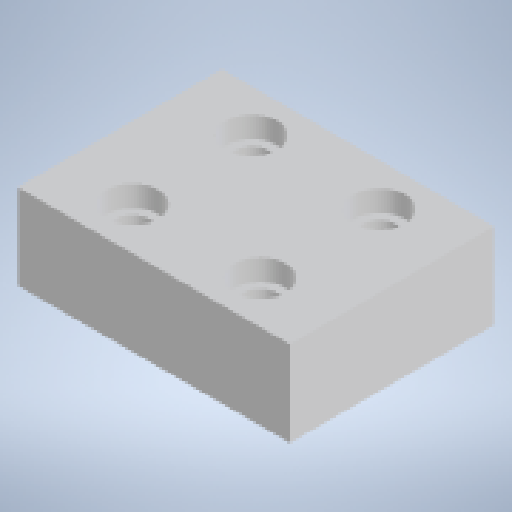
# Autodesk Inventor part: WristMotorTensioner
Saved by Autodesk Inventor 2024 (Build 280153000, 153)
## iProperties
Created: 2024-02-06
Part Number: WristMotorTensioner
Material: Generic
Document SubType Name: Modeling
Designer: Irwin
Density: 1 g/cm^3
Appearance: Default
Author: Irwin
Autodesk Inventor part; units mm, degrees
ref_plane "YZ Plane" through (0, 0, 0) normal (1, 0, 0) x (0, 1, 0)
ref_plane "XZ Plane" through (0, 0, 0) normal (0, 1, 0) x (-1, 0, 0)
ref_plane "XY Plane" through (0, 0, 0) normal (0, 0, 1) x (1, 0, 0)
sketch "Sketch1" plane through (0, 0, 0) normal (0, 1, 0) x (-1, 0, 0)
  line L0 (0, 0) -> (-32, 0)
  line L1 (-32, 0) -> (-32, -24)
  line L2 (-32, -24) -> (0, -24)
  line L3 (0, -24) -> (0, 0)
  circle A0 centre (-8.5, -19) radius 2
  circle A1 centre (-23.5, -19) radius 2
  circle A2 centre (-23.5, -5) radius 2
  circle A3 centre (-8.5, -5) radius 2
  line L4 (-16, -24) -> (-16, 0) construction
  line L5 (0, -12) -> (-32, -12) construction
  dimension "d0" = 32
  dimension "d1" = 24
  dimension "x" = 4
  dimension "d3" = 4
  dimension "d4" = 4
  dimension "d5" = 4
  dimension "d6" = 15
  dimension "d7" = 7.5
  dimension "d8" = 14
  dimension "d9" = 7
  constraints: 12 end point, 4 centre point, 4 midpoint, 2 horizontal alignment, 2 parallel, 2 vertical alignment, 1 horizontal, 1 perpendicular
  measures "d0" distance of L2.end L1.end
  measures "d1" distance of L0.end L1.end
  measures "x" diameter of A0
  measures "d3" diameter of A1
  measures "d4" diameter of A2
  measures "d5" diameter of A3
  measures "d6" distance of A1.centre A0.centre
  measures "d7" distance from line of A1.centre L4
  measures "d8" distance of A2.centre A1.centre
  measures "d9" distance from line of A2.centre L5
extrude "Extrusion1" add sketch "Sketch1" along normal blind 10
sketch "Sketch2" plane through (0, 10, 0) normal (0, 1, 0) x (1, 0, 0)
  circle A0 centre (23.5, 5) radius 2 projected
  circle A1 centre (8.5, 19) radius 2 projected
  circle A2 centre (23.5, 19) radius 2 projected
  circle A3 centre (8.5, 5) radius 2 projected
  circle A4 centre (8.5, 19) radius 3
  circle A5 centre (23.5, 19) radius 3
  circle A6 centre (8.5, 5) radius 3
  circle A7 centre (23.5, 5) radius 3
  point P0 (0, 0)
  dimension "d12" = 6
  dimension "d13" = 6
  dimension "d14" = 6
  dimension "d15" = 6
  constraints: 4 centre point, 4 coincident
  measures "d12" diameter of A4
  measures "d13" diameter of A5
  measures "d14" diameter of A6
  measures "d15" diameter of A7
extrude "Extrusion2" cut sketch "Sketch2" against normal blind 2.5 contours A3 | A4 | A5 | A6 | A7
equation "\"d3\" = x"
equation "\"d4\" = x"
equation "\"d5\" = x"
body "Solid1"
